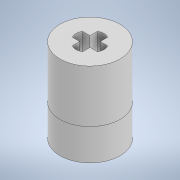
# Autodesk Inventor part: Servo_stycke
Saved by Autodesk Inventor 2021 (Build 250183000, 183)
## iProperties
Created: 2024-04-23
Part Number: Servo_stycke
Material: Generic
Document SubType Name: Modeling
Designer: 23adrdam
Density: 1 g/cm^3
Appearance: Default
Author: 23adrdam
Autodesk Inventor part; units mm, degrees
ref_plane "YZ Plane" through (0, 0, 0) normal (1, 0, 0) x (0, 1, 0)
ref_plane "XZ Plane" through (0, 0, 0) normal (0, 1, 0) x (-1, 0, 0)
ref_plane "XY Plane" through (0, 0, 0) normal (0, 0, 1) x (1, 0, 0)
sketch "Sketch1" plane through (0, 0, 0) normal (0, 1, 0) x (-1, 0, 0)
  arc A0 (0, 3.5698) -> (-0.36, 3.2098) centre (0, 3.2098) ccw
  arc A1 (0.36, 3.2098) -> (0, 3.5698) centre (0, 3.2098) ccw
  line L0 (0, 3.5698) -> (0, 3.5698)
  line L1 (-2.5242, 2.0151) -> (-1.7605, 1.2514)
  arc A2 (-2.0151, 2.5242) -> (-2.5242, 2.5242) centre (-2.2697, 2.2697) ccw
  line L2 (-2.5242, 2.5242) -> (-2.5242, 2.5242)
  arc A3 (-2.5242, 2.5242) -> (-2.5242, 2.0151) centre (-2.2697, 2.2697) ccw
  line L3 (-3.2098, 0.36) -> (-2.1298, 0.36)
  arc A4 (-2.1298, 0.36) -> (-2.1298, -0.36) centre (0, 0) ccw
  line L4 (-3.2098, -0.36) -> (-2.1298, -0.36)
  arc A5 (-3.2098, 0.36) -> (-3.5698, 0) centre (-3.2098, 0) ccw
  line L5 (-3.5698, 0) -> (-3.5698, 0)
  arc A6 (-3.5698, 0) -> (-3.2098, -0.36) centre (-3.2098, 0) ccw
  line L6 (-2.5242, -2.0151) -> (-1.7605, -1.2514)
  arc A7 (-2.5242, -2.0151) -> (-2.5242, -2.5242) centre (-2.2697, -2.2697) ccw
  line L7 (-2.5242, -2.5242) -> (-2.5242, -2.5242)
  arc A8 (-2.5242, -2.5242) -> (-2.0151, -2.5242) centre (-2.2697, -2.2697) ccw
  line L8 (-2.0151, -2.5242) -> (-1.2514, -1.7605)
  arc A9 (-1.7605, -1.2514) -> (-1.2514, -1.7605) centre (0, 0) ccw
  line L9 (-0.36, -3.2098) -> (-0.36, -2.1298)
  arc A10 (-0.36, -2.1298) -> (0.36, -2.1298) centre (0, 0) ccw
  arc A11 (-0.36, -3.2098) -> (0, -3.5698) centre (0, -3.2098) ccw
  line L10 (0, -3.5698) -> (0, -3.5698)
  arc A12 (0, -3.5698) -> (0.36, -3.2098) centre (0, -3.2098) ccw
  line L11 (0.36, -3.2098) -> (0.36, -2.1298)
  line L12 (2.0151, -2.5242) -> (1.2514, -1.7605)
  arc A13 (1.2514, -1.7605) -> (1.7605, -1.2514) centre (0, 0) ccw
  arc A14 (2.0151, -2.5242) -> (2.5242, -2.5242) centre (2.2697, -2.2697) ccw
  line L13 (2.5242, -2.5242) -> (2.5242, -2.5242)
  arc A15 (2.5242, -2.5242) -> (2.5242, -2.0151) centre (2.2697, -2.2697) ccw
  line L14 (2.5242, -2.0151) -> (1.7605, -1.2514)
  line L15 (3.2098, -0.36) -> (2.1298, -0.36)
  arc A16 (2.1298, -0.36) -> (2.1298, 0.36) centre (0, 0) ccw
  line L16 (3.2098, 0.36) -> (2.1298, 0.36)
  arc A17 (3.2098, -0.36) -> (3.5698, 0) centre (3.2098, 0) ccw
  line L17 (3.5698, 0) -> (3.5698, 0)
  arc A18 (3.5698, 0) -> (3.2098, 0.36) centre (3.2098, 0) ccw
  line L18 (2.5242, 2.0151) -> (1.7605, 1.2514)
  arc A19 (1.7605, 1.2514) -> (1.2514, 1.7605) centre (0, 0) ccw
  arc A20 (2.5242, 2.0151) -> (2.5242, 2.5242) centre (2.2697, 2.2697) ccw
  line L19 (2.5242, 2.5242) -> (2.5242, 2.5242)
  arc A21 (2.5242, 2.5242) -> (2.0151, 2.5242) centre (2.2697, 2.2697) ccw
  line L20 (2.0151, 2.5242) -> (1.2514, 1.7605)
  line L21 (0.36, 3.2098) -> (0.36, 2.1298)
  arc A22 (0.36, 2.1298) -> (-0.36, 2.1298) centre (0, 0) ccw
  line L22 (-2.0151, 2.5242) -> (-1.2514, 1.7605)
  arc A23 (-1.2514, 1.7605) -> (-1.7605, 1.2514) centre (0, 0) ccw
  circle A24 centre (0, 0) radius 2.16
  line L23 (-0.36, 3.2098) -> (-0.36, 2.1298)
  circle A25 centre (0, 0) radius 5.7281
  point P0 (-0.36, 3.5698)
  point P1 (0.36, 3.5698)
  point P2 (-2.0323, 2.0323)
  point P3 (-2.7788, 2.2697)
  point P4 (-2.2697, 2.7788)
  point P5 (-3.5698, 0.36)
  point P6 (-2.8742, 0)
  point P7 (-3.5698, -0.36)
  point P8 (-2.7788, -2.2697)
  point P9 (-2.0323, -2.0323)
  point P10 (-2.2697, -2.7788)
  point P11 (-0.36, -3.5698)
  point P12 (0, -2.8742)
  point P13 (0.36, -3.5698)
  point P14 (2.2697, -2.7788)
  point P15 (2.0323, -2.0323)
  point P16 (2.7788, -2.2697)
  point P17 (3.5698, -0.36)
  point P18 (2.8742, 0)
  point P19 (3.5698, 0.36)
  point P20 (2.7788, 2.2697)
  point P21 (2.2697, 2.7788)
  point P22 (2.0323, 2.0323)
  point P23 (0, 2.8742)
  point P24 (-2.5242, 2.5242)
  point P25 (0, 3.5698)
  point P26 (1.2514, 1.7605)
  point P27 (2.5242, 2.5242)
  point P28 (1.7605, -1.2514)
  point P29 (2.5242, -2.5242)
  point P30 (0, -3.5698)
  point P31 (-1.2514, -1.7605)
  point P32 (-2.5242, -2.5242)
  point P33 (-3.5698, 0)
  point P34 (-1.7605, 1.2514)
  dimension "d2" = 4.32
  dimension "d3" = 0.72
  dimension "d4" = 1.44
  dimension "d5" = 1.44
  dimension "d6" = 0.36
  dimension "d7" = 360
  constraints: 50 point on circle, 48 end point, 32 point on line, 26 centre point, 4 tangent, 2 coincident, 2 concentric, 1 horizontal, 1 vertical, 145 other
  measures "d2" diameter of A24
  measures "d3" distance between parallel lines of L23 L21
  measures "d4" distance of point (-0.36, 3.57) L23.end
  measures "d5" distance of point (0.36, 3.57) L21.end
  measures "d6" radius of A0
extrude "Extrusion1" add sketch "Sketch1" along normal blind 5
sketch "Sketch2" plane through (0, 5, 0) normal (0, 1, 0) x (1, 0, 0)
  circle A0 centre (0, 0) radius 5.7281
  constraints: 1 centre point, 1 coincident
extrude "Extrusion2" add sketch "Sketch2" along normal blind 1
sketch "Sketch7" plane through (0, 6, 0) normal (0, 1, 0) x (1, 0, 0)
  line L0 (2.3926, -0.9756) -> (2.3926, 0.9756)
  line L1 (2.3926, 0.9756) -> (0.9755, 0.9755)
  line L2 (0.9755, 0.9755) -> (0.9754, 2.3926)
  line L3 (0.9754, 2.3926) -> (-0.9756, 2.3926)
  arc A0 (0.9754, 2.3926) -> (-0.9756, 2.3926) centre (0, 0.8054) ccw
  arc A1 (2.3926, -0.9756) -> (2.3926, 0.9756) centre (0.8054, 0) ccw
  line L4 (2.3926, -0.9756) -> (0.9755, -0.9756)
  line L5 (0.9755, -0.9756) -> (0.9756, -2.3926)
  line L6 (0.9756, -2.3926) -> (-0.9755, -2.3926)
  arc A2 (-0.9755, -2.3926) -> (0.9756, -2.3926) centre (0, -0.8054) ccw
  line L7 (-0.9756, 2.3926) -> (-0.9756, 0.9756)
  line L8 (-0.9755, -2.3926) -> (-0.9756, -0.9755)
  line L9 (-0.9756, 0.9756) -> (-2.3926, 0.9756)
  line L10 (-2.3926, 0.9756) -> (-2.3925, -0.9755)
  line L11 (-2.3925, -0.9755) -> (-0.9756, -0.9755)
  arc A3 (-2.3926, 0.9756) -> (-2.3925, -0.9755) centre (-0.8054, 0) ccw
  circle A4 centre (0, 0) radius 5.728
  dimension "d29" = 1.951
  dimension "d32" = 1.9511
  dimension "d34" = 0.9756
  dimension "d31" = 1.4171
  dimension "d30" = 1.417
  dimension "d33" = 2.5838
  dimension "d28" = 1.863
  dimension "d27" = 1.863
  dimension "d25" = 1.417
  dimension "d24" = 1.9511
  dimension "d23" = 1.863
  dimension "d26" = 1.417
  dimension "d21" = 2.5838
  dimension "d20" = 1.9511
  dimension "d19" = 1.863
  dimension "d18" = 2.3925
  dimension "d17" = 2.3925
  dimension "d22" = 1.417
  dimension "d16" = 1.417
  dimension "d15" = 11.456
  constraints: 24 end point, 8 point on circle, 7 perpendicular, 6 coincident, 5 centre point, 2 horizontal, 2 vertical
  measures "d29" distance of L2.end L3.end
  measures "d32" distance of L0.start L0.end
  measures "d34" vertical distance of point (0, 0) L0.start
  measures "d31" distance of L0.end L1.end
  measures "d30" distance of L1.end L2.end
  measures "d33" distance of L0.start point (0, 0)
  measures "d28" radius of A0
  measures "d27" radius of A1
  measures "d25" distance of L4.end L5.end
  measures "d24" distance of L5.end L6.end
  measures "d23" radius of A2
  measures "d26" distance of L0.start L4.end
  measures "d21" distance of L10.end point (0, 0)
  measures "d20" distance of L9.end L10.end
  measures "d19" radius of A3
  measures "d18" distance from line of L3 point (0, 0)
  measures "d17" distance from line of L10 point (0, 0)
  measures "d22" distance of L7.end L9.end
  measures "d16" distance of L6.end L8.end
  measures "d15" diameter of A4
extrude "Extrusion4" add sketch "Sketch7" along normal blind 10
body "Solid1"
